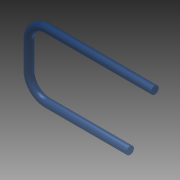
# Autodesk Inventor part: Water_tube
Saved by Autodesk Inventor 2015 (Build 190159000, 159)
## iProperties
Created: 2015-08-22
Part Number: Water_tube
Material: Water
Document SubType Name: Modeling
Designer: Kyle
Density: 0.9983 g/cm^3
Appearance: Tropical Blue
Author: Kyle
Autodesk Inventor part; units mm, degrees
ref_plane "YZ Plane" through (0, 0, 0) normal (1, 0, 0) x (0, 1, 0)
ref_plane "XZ Plane" through (0, 0, 0) normal (0, 1, 0) x (-1, 0, 0)
ref_plane "XY Plane" through (0, 0, 0) normal (0, 0, 1) x (1, 0, 0)
sketch "Sketch1" plane through (0, 0, 0) normal (0, 0, 1) x (1, 0, 0)
  line L0 (0, 2.159) -> (0, -2.159)
  line L1 (0, -2.159) -> (-61.595, -2.159)
  line L2 (0, 2.159) -> (-61.595, 2.159)
  line L3 (-61.595, -38.6842) -> (-14.4526, -38.6842)
  line L4 (-70.231, -13.1699) -> (-70.231, -23.3299)
  line L5 (-74.549, -13.1699) -> (-74.549, -23.3299)
  line L6 (-70.231, -13.1699) -> (-70.231, -2.159)
  line L7 (-70.231, -2.159) -> (-61.595, -2.159)
  line L8 (-61.595, 2.159) -> (-74.549, 2.159)
  line L9 (-74.549, 2.159) -> (-74.549, -13.1699)
  line L10 (-74.549, -23.3299) -> (-74.549, -38.6842)
  line L11 (-74.549, -38.6842) -> (-61.595, -38.6842)
  line L12 (-14.4526, -34.3662) -> (-14.4526, -36.5252)
  line L13 (-14.4526, -36.5252) -> (-14.4526, -38.6842)
  line L14 (-14.4526, -34.3662) -> (-70.231, -34.3662)
  line L15 (-70.231, -34.3662) -> (-70.231, -23.3299)
  point P0 (0, 0)
  point P1 (0, 0)
  point P2 (-61.595, 0)
  point P3 (-72.39, -18.2499)
  point P4 (-72.39, -13.1699)
  point P5 (-72.39, -23.3299)
  dimension "d0" = 61.595
  dimension "d1" = 18.2499
  dimension "d2" = 10.795
  dimension "d3" = 5.08
  dimension "d4" = 5.08
  dimension "d8" = 2.159
  dimension "d9" = 2.159
  dimension "d14" = 2.159
  dimension "d15" = 2.159
  dimension "d34" = 2.159
  dimension "d35" = 47.1424
  dimension "d36" = 36.5252
  constraints: 32 end point, 6 vertical, 5 horizontal, 4 perpendicular, 1 coincident, 1 collinear, 1 point on line
  measures "d0" distance of point (-61.595, 0) point (0, 0)
  measures "d1" vertical distance of point (-72.39, -18.25) point (-61.595, 0)
  measures "d2" horizontal distance of point (-72.39, -18.25) point (-61.595, 0)
  measures "d3" distance of point (-72.39, -18.25) point (-72.39, -13.17)
  measures "d4" distance of point (-72.39, -23.33) point (-72.39, -18.25)
  measures "d8" distance of point (0, 0) L0.start
  measures "d9" distance of point (0, 0) L0.end
  measures "d14" distance from line of point (-72.39, -13.17) L4
  measures "d15" distance from line of L5 point (-72.39, -13.17)
  measures "d34" distance of L3.end L12.end
  measures "d35" distance of L3.start L3.end
  measures "d36" vertical distance of L12.end point (0, 0)
extrude "Extrusion1" add sketch "Sketch1" along normal blind 4.318
fillet "Fillet10" radius 12.7 2 edges at (-74.549, 2.159, 2.159) (-74.549, -38.6842, 2.159)
fillet "Fillet11" radius 8.382 2 edges at (-70.231, -34.3662, 2.159) (-70.231, -2.159, 2.159)
fillet "Fillet12" radius 2.159 20 edges at (-70.8293, -1.5607, 0) (-74.549, -18.2499, 0) (-70.8293, -34.9645, 0) (-38.0238, -38.6842, 0) (-30.7975, 2.159, 0) (-70.8293, -1.5607, 4.318) (-74.549, -18.2499, 4.318) (-70.8293, -34.9645, 4.318) (-38.0238, -38.6842, 4.318) (-61.722, 2.159, 4.318) (-67.776, -31.9112, 4.318) (-70.231, -18.2499, 4.318) (-67.776, -4.614, 4.318) (-30.7975, -2.159, 4.318) (-38.1508, -34.3662, 4.318) (-67.776, -31.9112, 0) (-70.231, -18.2499, 0) (-67.776, -4.614, 0) (-30.7975, -2.159, 0) (-38.1508, -34.3662, 0)
sketch "Sketch5" plane through (0, 0, 2.159) normal (1, 0, 0) x (0, 0, -1)
  circle A0 centre (0, 0) radius 2.159
  point P0 (2.159, 0)
  constraints: 1 horizontal alignment, 2 other
extrude "Extrusion5" cut sketch "Sketch5" against normal blind 1.27
sketch "Sketch6" plane through (-14.4526, -36.5252, 2.159) normal (1, 0, 0) x (0, 0, -1)
  circle A0 centre (0, 0) radius 2.1591
  point P0 (2.159, 36.5252)
  constraints: 1 centre point
extrude "Extrusion6" cut sketch "Sketch6" against normal blind 0.7874
body "Solid1"
